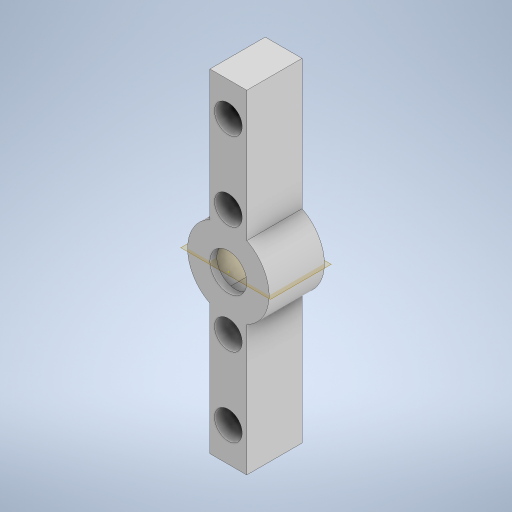
# Autodesk Inventor part: Lead Nut Holder
Saved by Autodesk Inventor 2024 (Build 280153000, 153)
## iProperties
Created: 2024-01-10
Part Number: Lead Nut Holder
Material: Generic
Document SubType Name: Modeling
Designer: aidan
Density: 1 g/cm^3
Appearance: Default
Author: aidan
Autodesk Inventor part; units mm, degrees
ref_plane "YZ Plane" through (0, 0, 0) normal (1, 0, 0) x (0, 1, 0)
ref_plane "XY Plane" through (0, 0, 0) normal (0, 0, 1) x (1, 0, 0)
sketch "Sketch1" plane through (0, 0, 0) normal (0, 0, 1) x (1, 0, 0)
  circle A0 centre (0, 0) radius 3.175
  circle A1 centre (0, 0) radius 6.35
  dimension "d0" = 6.35
  dimension "d1" = 12.7
  constraints: 2 centre point, 2 coincident
  measures "d0" diameter of A0
  measures "d1" diameter of A1
extrude "Extrusion1" add sketch "Sketch1" along normal blind 5.9531
thread "Thread1" size "1/4-20 UNC" class "2B" standard "ANSI Unified Screw Threads" full length
sketch "Sketch2" plane through (0, 0, 5.9531) normal (0, 0, 1) x (1, 0, 0)
  circle A0 centre (0, 0) radius 6.35 projected
  line L0 (-6.35, 0) -> (-3.175, 5.4993)
  line L1 (-3.175, 5.4993) -> (3.175, 5.4993)
  line L2 (3.175, 5.4993) -> (6.35, 0)
  line L3 (6.35, 0) -> (3.175, -5.4993)
  line L4 (3.175, -5.4993) -> (-3.175, -5.4993)
  line L5 (-3.175, -5.4993) -> (-6.35, 0)
  point P0 (-3.175, -5.4993)
  point P1 (-3.175, -5.4993)
  constraints: 12 end point, 1 coincident, 15 other
extrude "Extrusion2" cut sketch "Sketch2" against normal blind 11.1125 contours L2 A0 | A0 L3 | L1 A0 | A0 L4 | L0 A0 | A0 L5
sketch "Sketch3" plane through (0, 0, 5.9531) normal (0, 0, 1) x (1, 0, 0)
  circle A0 centre (0, 0) radius 7.0182
  line L0 (3.175, 5.4993) -> (-3.175, 5.4993) projected
  line L1 (3.175, 5.4993) -> (-3.175, 5.4993)
  line L2 (-3.175, 5.4993) -> (-3.175, 19.05)
  line L3 (-3.175, 19.05) -> (3.175, 19.05)
  line L4 (3.175, 19.05) -> (3.175, 5.4993)
  line L5 (-3.175, -5.4993) -> (3.175, -5.4993) projected
  line L6 (-3.175, -5.4993) -> (3.175, -5.4993)
  line L7 (3.175, -5.4993) -> (3.175, -19.05)
  line L8 (3.175, -19.05) -> (-3.175, -19.05)
  line L9 (-3.175, -19.05) -> (-3.175, -5.4993)
  circle A1 centre (0, 15.24) radius 1.3093
  circle A2 centre (0, -15.24) radius 1.5457
  point P0 (-3.175, 6.2589)
  point P1 (-3.175, -6.2589)
  point P2 (3.175, -6.2589)
  point P3 (3.175, 6.2589)
  dimension "d9" = 38.1
  dimension "d10" = 15.24
  dimension "d11" = 15.24
  constraints: 16 end point, 4 parallel, 3 centre point, 2 horizontal, 2 perpendicular, 1 coincident, 1 collinear, 1 point on line
  measures "d9" distance of L8.end L2.end
  measures "d10" distance of point (0, 0) A1.centre
  measures "d11" distance of A2.centre point (0, 0)
sketch "Sketch4" plane through (0, 0, 0) normal (0, 0, -1) x (-1, 0, 0)
  line L0 (3.175, 5.4993) -> (-3.175, 5.4993) projected
  line L1 (-3.175, 5.4993) -> (-6.35, 0) projected
  line L2 (-6.35, 0) -> (-3.175, -5.4993) projected
  line L3 (-3.175, -5.4993) -> (3.175, -5.4993) projected
  line L4 (3.175, -5.4993) -> (6.35, 0) projected
  line L5 (6.35, 0) -> (3.175, 5.4993) projected
  circle A0 centre (0, 0) radius 3.175 projected
extrude "Extrusion3" add sketch "Sketch4" along normal blind 15.875
extrude "Extrusion4" add sketch "Sketch3" against normal blind 6.35
sketch "Sketch5" plane through (0, 0, -15.875) normal (0, 0, -1) x (-1, 0, 0)
  line L0 (-3.175, 5.4993) -> (-6.35, 0) projected
  line L1 (-6.35, 0) -> (-3.175, -5.4993) projected
  line L2 (-3.175, -5.4993) -> (3.175, -5.4993) projected
  line L3 (3.175, -5.4993) -> (6.35, 0) projected
  line L4 (6.35, 0) -> (3.175, 5.4993) projected
  line L5 (3.175, 5.4993) -> (-3.175, 5.4993) projected
  circle A0 centre (0, 0) radius 3.175 projected
extrude "Extrusion5" cut sketch "Sketch5" against normal blind 20.6375
sketch "Sketch6" plane through (0, 0, -0.3969) normal (0, 0, -1) x (-1, 0, 0)
  circle A0 centre (0, 0) radius 3.175 projected
extrude "Extrusion6" cut sketch "Sketch6" against normal blind 92.075
sketch "Sketch7" plane through (0, 0, -0.3969) normal (0, 0, -1) x (-1, 0, 0)
  circle A0 centre (0, 15.24) radius 1.3093 projected
  circle A1 centre (0, -15.24) radius 1.5457 projected
  line L0 (3.175, -19.05) -> (3.175, -6.2589) projected
  arc A2 (3.175, -6.2589) -> (3.175, 6.2589) centre (0, 0) ccw projected
  line L1 (3.175, 6.2589) -> (3.175, 19.05) projected
  line L2 (3.175, 19.05) -> (-3.175, 19.05) projected
  line L3 (-3.175, 19.05) -> (-3.175, 6.2589) projected
  arc A3 (-3.175, 6.2589) -> (-3.175, -6.2589) centre (0, 0) ccw projected
  line L4 (-3.175, -6.2589) -> (-3.175, -19.05) projected
  line L5 (-3.175, -19.05) -> (3.175, -19.05) projected
  line L6 (-3.175, -5.4993) -> (3.175, -5.4993) projected
  line L7 (-6.35, 0) -> (-3.175, -5.4993) projected
  line L8 (-3.175, 5.4993) -> (-6.35, 0) projected
  line L9 (3.175, 5.4993) -> (-3.175, 5.4993) projected
  line L10 (6.35, 0) -> (3.175, 5.4993) projected
  line L11 (3.175, -5.4993) -> (6.35, 0) projected
extrude "Extrusion7" add sketch "Sketch7" along normal blind 3.175
sketch "Sketch8" plane through (0, 0, 5.9531) normal (0, 0, 1) x (1, 0, 0)
  circle A0 centre (0, 15.24) radius 1.3093 projected
  circle A1 centre (0, 15.24) radius 2.3813
  circle A2 centre (0, 8.0246) radius 2.3812
  circle A3 centre (0, -7.1942) radius 2.7326
  circle A4 centre (0, -15.24) radius 1.5457 projected
  circle A5 centre (0, -15.24) radius 2.3813
  point P0 (0, 0)
  dimension "d22" = 4.7625
  dimension "d23" = 4.7625
  dimension "d24" = 4.7625
  constraints: 4 centre point, 2 coincident
  measures "d22" diameter of A1
  measures "d23" diameter of A2
  measures "d24" diameter of A5
extrude "Extrusion8" cut sketch "Sketch8" against normal blind 41.275 contours A1 | A2 | A3 | A4 | A5
sketch "Sketch9" plane through (0, 0, 4.7625) normal (0, 0, -1) x (-1, 0, 0)
  line L0 (3.175, -5.4993) -> (2.1434, -5.4993) projected
  line L1 (-2.1434, -5.4993) -> (-3.175, -5.4993) projected
  line L2 (2.1434, -5.4993) -> (-2.1434, -5.4993)
  line L3 (2.1434, -5.4993) -> (1.8696, -3.3678)
  line L4 (1.8696, -3.3678) -> (-1.765, -3.8347)
  line L5 (-1.765, -3.8347) -> (-2.1434, -5.4993)
  point P0 (0, 0)
  constraints: 8 end point, 1 horizontal, 1 perpendicular
extrude "Extrusion9" add sketch "Sketch9" along normal up to surface (8.3344 mm away)
sketch "Sketch10" plane through (0, 0, -3.5719) normal (0, 0, -1) x (-1, 0, 0)
  line L0 (6.35, 0) -> (3.175, -5.4993) projected
  line L1 (6.35, 0) -> (3.175, -5.4993)
  line L2 (3.175, -5.4993) -> (-3.175, -5.4993)
  line L3 (-3.175, -5.4993) -> (-6.35, 0)
  line L4 (-6.35, 0) -> (-3.175, 5.4993)
  line L5 (-3.175, 5.4993) -> (3.175, 5.4993)
  line L6 (3.175, 5.4993) -> (6.35, 0)
  point P0 (0, 0)
  point P1 (0, 0)
  constraints: 12 end point, 1 coincident, 13 other
sketch "Sketch11" plane through (0, 0, -3.5719) normal (0, 0, -1) x (-1, 0, 0)
  line L0 (2.1434, -5.4993) -> (-2.1434, -5.4993) projected
  circle A0 centre (0, -9.3093) radius 2.3813
  circle A1 centre (0, 9.3093) radius 2.3813
  line L1 (-3.175, 5.4993) -> (3.175, 5.4993) projected
  point P0 (0, 0)
  point P1 (0, -7.1942)
  point P2 (0, -5.4993)
  dimension "d32" = 4.7625
  dimension "d33" = 3.81
  dimension "d34" = 4.7625
  dimension "d35" = 3.81
  constraints: 2 centre point, 1 midpoint
  measures "d32" diameter of A0
  measures "d33" distance of point (0, -5.499) A0.centre
  measures "d34" diameter of A1
  measures "d35" distance from line of L1 A1.centre
extrude "Extrusion10" cut sketch "Sketch11" against normal blind 46.0375
sketch "Sketch12" plane through (3.175, 6.2589, 5.9531) normal (1, 0, 0) x (0, 0, -1)
  point P0 (5.9531, -6.2589)
sketch "Sketch13" plane through (0, 0, 5.9531) normal (0, 0, 1) x (1, 0, 0)
  arc A0 (2.293, 8.6669) -> (-2.293, 8.6669) centre (0, 9.3093) ccw projected
  circle A1 centre (0, 9.3093) radius 2.3812
  arc A2 (-2.293, 8.6669) -> (2.293, 8.6669) centre (0, 8.0246) ccw
  arc A3 (2.2956, -8.6765) -> (-2.2956, -8.6765) centre (0, -7.1942) ccw projected
  arc A4 (2.2956, -8.6765) -> (-2.2956, -8.6765) centre (0, -7.1942) ccw
  arc A5 (-2.2956, -8.6765) -> (2.2956, -8.6765) centre (0, -9.3093) ccw projected
  circle A6 centre (0, -9.3093) radius 2.3812
  point P0 (0, 0)
  point P1 (-2.2956, -8.6765)
  constraints: 4 centre point, 4 point on circle, 2 coincident
extrude "Extrusion11" add sketch "Sketch13" against normal up to surface (9.525 mm away) contours A2 A1 | A6 A3
extrude "Extrusion12" cut sketch "Sketch10" against normal up to surface (8.3344 mm away)
sketch "Sketch14" plane through (0, 0, -3.5719) normal (0, 0, -1) x (-1, 0, 0)
  line L0 (3.175, -19.05) -> (3.175, -6.2589) projected
  line L1 (-3.175, -19.05) -> (3.175, -19.05) projected
  line L2 (3.175, -11.8753) -> (-3.175, -11.8753)
  line L3 (-3.175, -11.8753) -> (-3.175, -19.05)
  line L4 (-3.175, -19.05) -> (3.175, -19.05)
  line L5 (3.175, -19.05) -> (3.175, -11.8753)
  line L6 (3.175, 19.05) -> (3.175, 6.2589) projected
  line L7 (3.175, 12.0286) -> (-3.175, 12.0286)
  line L8 (-3.175, 12.0286) -> (-3.175, 19.05)
  line L9 (-3.175, 19.05) -> (3.175, 19.05)
  line L10 (3.175, 19.05) -> (3.175, 12.0286)
  point P0 (0, 0)
  constraints: 16 end point, 4 parallel, 3 point on line, 2 horizontal, 2 perpendicular
extrude "Extrusion13" add sketch "Sketch14" against normal up to surface (9.525 mm away)
sketch "Sketch15" plane through (0, 0, 5.9531) normal (0, 0, 1) x (1, 0, 0)
  point P0 (0, 0)
sketch "Sketch16" plane through (-3.175, 19.05, 5.9531) normal (0, 1, 0) x (1, 0, 0)
  line L0 (6.35, 0) -> (0, 0) projected
  line L1 (6.35, 0) -> (6.35, 9.525) projected
  line L2 (0, 9.525) -> (6.35, 9.525) projected
  line L3 (0, 0) -> (0, 9.525) projected
  line L4 (0, 0) -> (6.35, 0) projected
  line L5 (0, 0) -> (0, 9.525) projected
  line L6 (6.35, 9.525) -> (0, 9.525) projected
  line L7 (6.35, 0) -> (6.35, 9.525) projected
  point P0 (3.175, 5.9531)
extrude "Extrusion14" add sketch "Sketch16" along normal blind 9.652
sketch "Sketch17" plane through (-3.175, -19.05, 5.9531) normal (0, -1, 0) x (1, 0, 0)
  line L0 (0, 0) -> (6.35, 0) projected
  line L1 (0, 0) -> (0, -9.525) projected
  line L2 (6.35, -9.525) -> (0, -9.525) projected
  line L3 (6.35, 0) -> (6.35, -9.525) projected
  point P0 (3.175, -5.9531)
extrude "Extrusion15" add sketch "Sketch17" along normal blind 9.652
sketch "Sketch18" plane through (0, 0, -3.5719) normal (0, 0, -1) x (-1, 0, 0)
  circle A0 centre (0, 22.86) radius 2.3812
  circle A1 centre (0, -22.86) radius 2.3813
  point P0 (0, 0)
  dimension "d48" = 4.7625
  dimension "d49" = 4.7625
  dimension "d50" = 22.86
  dimension "d51" = 22.86
  constraints: 2 centre point
  measures "d48" diameter of A0
  measures "d49" diameter of A1
  measures "d50" distance of A0.centre point (0, 0)
  measures "d51" distance of point (0, 0) A1.centre
extrude "Extrusion16" cut sketch "Sketch18" against normal blind 18.923
body "Solid1"
